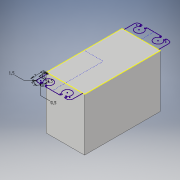
# Autodesk Inventor part: CH_01_0004_servo_update
Saved by Autodesk Inventor 2019 (Build 230136000, 136)
## iProperties
Created: 2022-02-28
Part Number: CH_01_0004_servo_update
Material: Generic
Document SubType Name: Modeling
Designer: Tomasz Krakowski
Density: 1 g/cm^3
Appearance: Default
Author: Tomasz Krakowski
Autodesk Inventor part; units mm, degrees
ref_plane "YZ Plane" through (0, 0, 0) normal (1, 0, 0) x (0, 1, 0)
ref_plane "XZ Plane" through (0, 0, 0) normal (0, 1, 0) x (-1, 0, 0)
ref_plane "XY Plane" through (0, 0, 0) normal (0, 0, 1) x (1, 0, 0)
sketch "Sketch1" plane through (0, 0, 0) normal (0, 1, 0) x (-1, 0, 0)
  line L0 (-10.25, 20.25) -> (10.25, 20.25)
  line L1 (10.25, 20.25) -> (10.25, -20.25)
  line L2 (10.25, -20.25) -> (-10.25, -20.25)
  line L3 (-10.25, -20.25) -> (-10.25, 20.25)
  line L4 (-10.25, 20.25) -> (10.25, -20.25) construction
  line L5 (10.25, 20.25) -> (-10.25, -20.25) construction
  point P0 (0, 0)
  dimension "d0" = 20.5
  dimension "d1" = 40.5
  constraints: 12 end point, 2 midpoint, 2 parallel, 1 horizontal, 1 perpendicular
  measures "d0" distance between parallel lines of L3 L1
  measures "d1" distance between parallel lines of L2 L0
extrude "Extrusion1" add sketch "Sketch1" along normal blind 28.3
sketch "Sketch2" plane through (0, 28.3, 0) normal (0, 1, 0) x (1, 0, 0)
  line L0 (-10.25, -20.25) -> (10.25, -20.25) projected
  line L1 (10.25, -20.25) -> (10.25, 20.25) projected
  line L2 (10.25, 20.25) -> (-10.25, 20.25) projected
  line L3 (-10.25, 20.25) -> (-10.25, -20.25) projected
  line L4 (0, 0) -> (-10.25, 0) construction
  arc A0 (-3.9773, -26.2541) -> (-6.4318, -25.9856) centre (-5, -24.25) ccw
  line L5 (-10.25, -20.25) -> (10.25, -20.25) construction
  line L6 (0, -20.25) -> (0, 0) construction
  line L7 (-6.25, -26.3713) -> (-6.25, -26.75)
  line L8 (-6.75, -27.25) -> (-7.75, -27.25)
  line L9 (-9.25, -25.75) -> (-9.25, -20.25)
  arc A1 (-9.25, -25.75) -> (-7.75, -27.25) centre (-7.75, -25.75) ccw
  line L10 (-4.25, -26.6995) -> (-4.25, -26.75)
  line L11 (-3.75, -27.25) -> (0, -27.25)
  line L12 (0, -27.25) -> (0, -20.25) construction
  arc A2 (-6.75, -27.25) -> (-6.25, -26.75) centre (-6.75, -26.75) ccw
  arc A3 (-4.25, -26.75) -> (-3.75, -27.25) centre (-3.75, -26.75) ccw
  arc A4 (-3.9773, -26.2541) -> (-4.25, -26.6995) centre (-3.75, -26.6995) ccw
  arc A5 (-6.25, -26.3713) -> (-6.4318, -25.9856) centre (-6.75, -26.3713) ccw
  arc A6 (6.4318, -25.9856) -> (3.9773, -26.2541) centre (5, -24.25) ccw
  line L13 (6.25, -26.3713) -> (6.25, -26.75)
  line L14 (6.75, -27.25) -> (7.75, -27.25)
  line L15 (9.25, -25.75) -> (9.25, -20.25)
  arc A7 (7.75, -27.25) -> (9.25, -25.75) centre (7.75, -25.75) ccw
  line L16 (4.25, -26.6995) -> (4.25, -26.75)
  line L17 (3.75, -27.25) -> (0, -27.25)
  arc A8 (6.25, -26.75) -> (6.75, -27.25) centre (6.75, -26.75) ccw
  arc A9 (3.75, -27.25) -> (4.25, -26.75) centre (3.75, -26.75) ccw
  arc A10 (4.25, -26.6995) -> (3.9773, -26.2541) centre (3.75, -26.6995) ccw
  arc A11 (6.4318, -25.9856) -> (6.25, -26.3713) centre (6.75, -26.3713) ccw
  arc A12 (-6.4318, 25.9856) -> (-3.9773, 26.2541) centre (-5, 24.25) ccw
  line L18 (-6.25, 26.3713) -> (-6.25, 26.75)
  line L19 (-6.75, 27.25) -> (-7.75, 27.25)
  line L20 (-9.25, 25.75) -> (-9.25, 20.25)
  arc A13 (-7.75, 27.25) -> (-9.25, 25.75) centre (-7.75, 25.75) ccw
  line L21 (-4.25, 26.6995) -> (-4.25, 26.75)
  line L22 (-3.75, 27.25) -> (0, 27.25)
  line L23 (0, 27.25) -> (0, 20.25) construction
  arc A14 (-6.25, 26.75) -> (-6.75, 27.25) centre (-6.75, 26.75) ccw
  arc A15 (-3.75, 27.25) -> (-4.25, 26.75) centre (-3.75, 26.75) ccw
  arc A16 (-4.25, 26.6995) -> (-3.9773, 26.2541) centre (-3.75, 26.6995) ccw
  arc A17 (-6.4318, 25.9856) -> (-6.25, 26.3713) centre (-6.75, 26.3713) ccw
  arc A18 (9.25, 25.75) -> (7.75, 27.25) centre (7.75, 25.75) ccw
  line L24 (4.25, 26.6995) -> (4.25, 26.75)
  arc A19 (3.9773, 26.2541) -> (4.25, 26.6995) centre (3.75, 26.6995) ccw
  arc A20 (4.25, 26.75) -> (3.75, 27.25) centre (3.75, 26.75) ccw
  arc A21 (3.9773, 26.2541) -> (6.4318, 25.9856) centre (5, 24.25) ccw
  line L25 (9.25, 25.75) -> (9.25, 20.25)
  line L26 (3.75, 27.25) -> (0, 27.25)
  line L27 (6.25, 26.3713) -> (6.25, 26.75)
  line L28 (6.75, 27.25) -> (7.75, 27.25)
  arc A22 (6.75, 27.25) -> (6.25, 26.75) centre (6.75, 26.75) ccw
  arc A23 (6.25, 26.3713) -> (6.4318, 25.9856) centre (6.75, 26.3713) ccw
  point P0 (-6.25, -26.1208)
  point P1 (-4.25, -26.3713)
  point P2 (6.25, -26.1208)
  point P3 (4.25, -26.3713)
  point P4 (-6.25, 26.1208)
  point P5 (-4.25, 26.3713)
  point P6 (4.25, 26.3713)
  point P7 (6.25, 26.1208)
  dimension "d4" = 1.5
  dimension "d5" = 7
  dimension "d6" = 4
  dimension "d7" = 4.5
  dimension "d8" = 2
  dimension "d9" = 3
  dimension "d10" = 1
  dimension "d11" = 2
  dimension "d12" = 0.5
  constraints: 59 symmetric about line, 56 point on circle, 48 end point, 24 centre point, 10 tangent, 9 point on line, 4 perpendicular, 3 equal radius, 2 collinear, 2 midpoint, 2 vertical, 18 other
  measures "d4" radius of A1
  measures "d5" distance from line of L8 L9.end
  measures "d6" vertical distance of A0.centre L9.end
  measures "d7" diameter of A0
  measures "d8" distance edge to line of A0 L9
  measures "d9" distance between parallel lines of L9 L7
  measures "d10" distance between parallel lines of L3 L9
  measures "d11" distance between parallel lines of L7 L10
  measures "d12" radius of A2
body "Solid1"
